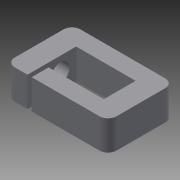
# Autodesk Inventor part: CounterWeightHook
Saved by Autodesk Inventor 2014 SP1 (Build 180222100, 222)
## iProperties
Created: 2017-02-25
Part Number: CounterWeightHook
Material: Generic
Document SubType Name: Modeling
Designer: danielsikar
Density: 1 g/cm^3
Appearance: Default
Author: danielsikar
Autodesk Inventor part; units mm, degrees
ref_plane "YZ Plane" through (0, 0, 0) normal (1, 0, 0) x (0, 1, 0)
ref_plane "XZ Plane" through (0, 0, 0) normal (0, 1, 0) x (-1, 0, 0)
ref_plane "XY Plane" through (0, 0, 0) normal (0, 0, 1) x (1, 0, 0)
sketch "Sketch1" plane through (0, 0, 0) normal (0, 0, 1) x (1, 0, 0)
  line L0 (0, 0) -> (24, 0)
  line L1 (24, 0) -> (24, 15.5)
  line L2 (24, 15.5) -> (0, 15.5)
  line L3 (0, 15.5) -> (0, 0)
  dimension "d0" = 24
  dimension "d1" = 15.5
  constraints: 8 end point, 2 parallel, 1 horizontal, 1 perpendicular
  measures "d0" distance of L2.end L1.end
  measures "d1" distance of L1.end L0.end
extrude "Extrusion1" add sketch "Sketch1" along normal blind 5
sketch "Sketch7" plane through (0, 0, 5) normal (0, 0, 1) x (1, 0, 0)
  line L0 (24, 15.5) -> (0, 15.5) projected
  line L1 (0, 15.5) -> (0, 0) projected
  line L2 (5, 11.5) -> (19, 11.5)
  line L3 (19, 11.5) -> (19, 4)
  line L4 (19, 4) -> (5, 4)
  line L5 (5, 4) -> (5, 11.5)
  point P0 (12, 11.5)
  point P1 (12, 15.5)
  point P2 (5, 7.75)
  point P3 (0, 7.75)
  dimension "d21" = 14
  dimension "d22" = 7.5
  constraints: 8 end point, 4 midpoint, 2 parallel, 1 horizontal, 1 horizontal alignment, 1 perpendicular, 1 vertical alignment
  measures "d21" distance of L3.end L4.end
  measures "d22" distance of L2.end L3.end
extrude "Extrusion7" cut sketch "Sketch7" against normal blind 5
sketch "Sketch8" plane through (0, 0, 0) normal (0, -1, 0) x (1, 0, 0)
  line L0 (0, 0) -> (24, 0) projected
  line L1 (5, 5) -> (5, 0) construction
  line L2 (5, 5) -> (6, 5)
  line L3 (6, 5) -> (6, 0)
  line L4 (6, 0) -> (5, 0)
  line L5 (5, 0) -> (5, 5)
  line L6 (0, 0) -> (0, 5) projected
  dimension "d34" = 5
  constraints: 8 end point, 2 parallel, 1 horizontal, 1 perpendicular, 1 point on line
  measures "d34" distance between parallel lines of L1 L6
extrude "Extrusion8" cut sketch "Sketch8" against normal blind 5
sketch "Sketch9" plane through (0, 0, 5) normal (0, 0, 1) x (1, 0, 0)
  line L0 (6, 4) -> (6, 0) projected
  line L1 (6, 0) -> (24, 0) projected
  line L2 (24, 0) -> (24, 15.5) projected
  line L3 (24, 15.5) -> (0, 15.5) projected
  line L4 (0, 15.5) -> (0, 0) projected
  line L5 (0, 0) -> (5, 0) projected
  line L6 (5, 0) -> (5, 11.5) projected
  line L7 (5, 11.5) -> (19, 11.5) projected
  line L8 (19, 11.5) -> (19, 4) projected
  line L9 (19, 4) -> (6, 4) projected
extrude "Extrusion9" add sketch "Sketch9" along normal blind 2
sketch "Sketch10" plane through (0, 0, 0) normal (-1, 0, 0) x (0, 0, 1)
  circle A0 centre (3.5, 7.75) radius 2.15
  dimension "d30" = 4.3
  constraints: 1 centre point
  measures "d30" diameter of A0
extrude "Extrusion10" cut sketch "Sketch10" against normal blind 5
fillet "Fillet2" radius 2 4 edges at (24, 0, 3.5) (24, 15.5, 3.5) (0, 0, 3.5) (0, 15.5, 3.5)
body "Solid1"
